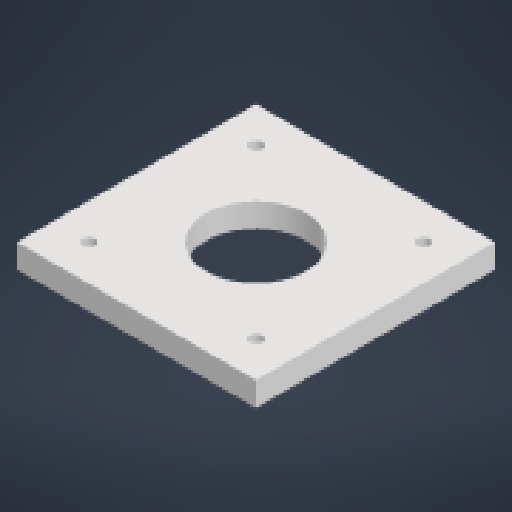
# Autodesk Inventor part: Bearing Plate
Saved by Autodesk Inventor 2023 (Build 270158000, 158)
## iProperties
Created: 2023-09-15
Part Number: Bearing Plate
Material: Generic
Document SubType Name: Modeling
Designer: Abhinav
Density: 1 g/cm^3
Appearance: Default
Author: Abhinav
Autodesk Inventor part; units mm, degrees
ref_plane "YZ Plane" through (0, 0, 0) normal (1, 0, 0) x (0, 1, 0)
ref_plane "XZ Plane" through (0, 0, 0) normal (0, 1, 0) x (-1, 0, 0)
ref_plane "XY Plane" through (0, 0, 0) normal (0, 0, 1) x (1, 0, 0)
sketch "Sketch1" plane through (0, 0, 0) normal (0, 1, 0) x (-1, 0, 0)
  circle A0 centre (-35, 35) radius 2.5
  circle A1 centre (35, -35) radius 2.5
  circle A2 centre (35, 35) radius 2.5
  circle A3 centre (-35, -35) radius 2.5
  line L0 (-35, -35) -> (35, -35) construction
  circle A4 centre (0, 0) radius 20.95
  line L1 (35, -35) -> (35, 35) construction
  line L2 (-35, 35) -> (-35, -35) construction
  line L3 (35, 35) -> (-35, 35) construction
  line L4 (-35, 35) -> (35, -35) construction
  line L5 (35, 35) -> (-35, -35) construction
  line L6 (50, 50) -> (-50, 50)
  line L7 (-50, 50) -> (-50, -50)
  line L8 (-50, -50) -> (50, -50)
  line L9 (50, -50) -> (50, 50)
  line L10 (50, 50) -> (-50, -50) construction
  line L11 (-50, 50) -> (50, -50) construction
  dimension "d4" = 41.9
  dimension "d5" = 70
  dimension "d6" = 70
  dimension "d7" = 5
  dimension "d8" = 100
  dimension "d9" = 100
  constraints: 24 end point, 5 centre point, 5 coincident, 4 midpoint, 4 parallel, 3 equal radius, 2 horizontal, 2 perpendicular
  measures "d4" diameter of A4
  measures "d5" distance of L0.end L0.start
  measures "d6" distance of L0.start L2.start
  measures "d7" diameter of A1
  measures "d8" distance of L8.end L7.end
  measures "d9" distance of L7.end L6.end
extrude "Extrusion1" add sketch "Sketch1" along normal blind 10
body "Solid1"
